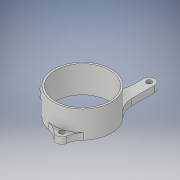
# Autodesk Inventor part: DPLX_P020_Camera Shroud Base_RevA
Saved by Autodesk Inventor 2018 (Build 220112000, 112)
## iProperties
Created: 2018-06-25
Part Number: DPLX_P020_Camera Shroud Base_RevA
Material: Generic
Document SubType Name: Modeling
Designer: Dplxuser
Density: 1 g/cm^3
Appearance: Default
Mass: 2.54454 g
Surface Area: 42.3669 cm^2
Volume: 2.54454 cm^3
Author: Dplxuser
Autodesk Inventor part; units mm, degrees
ref_plane "YZ Plane" through (0, 0, 0) normal (1, 0, 0) x (0, 1, 0)
ref_plane "XZ Plane" through (0, 0, 0) normal (0, 1, 0) x (-1, 0, 0)
ref_plane "XY Plane" through (0, 0, 0) normal (0, 0, 1) x (1, 0, 0)
sketch "Sketch2" plane through (0, 0, 0) normal (0, 1, 0) x (-1, 0, 0)
  circle A0 centre (-4.7625, 13.0048) radius 1.524 construction
  circle A1 centre (-25.3436, 13.0048) radius 6.35 construction
  circle A2 centre (-31.0168, 30.7721) radius 1.524 construction
  circle A3 centre (-31.0168, -20.6375) radius 1.524 construction
  line L0 (-38.1807, -25.4) -> (-38.1807, 35.5346) construction
  line L1 (-23.8528, -25.4) -> (-38.1807, -25.4) construction
  line L2 (-23.8528, 0) -> (-23.8528, -25.4) construction
  line L3 (0, 0) -> (-23.8528, 0) construction
  line L4 (0, 26.0096) -> (0, 0) construction
  line L5 (-23.8528, 26.0096) -> (0, 26.0096) construction
  line L6 (-23.8528, 26.0096) -> (-23.8528, 35.5346) construction
  line L7 (-38.1807, 35.5346) -> (-23.8528, 35.5346) construction
  point P0 (-23.8528, 13.0048)
  dimension "d3" = 3.048
  dimension "d4" = 12.7
  dimension "d5" = 90
  dimension "d6" = 23.8528
  dimension "d7" = 38.1807
  dimension "d8" = 26.0096
  dimension "d9" = 25.4
  dimension "d10" = 35.5346
  dimension "d11" = 0
  dimension "d12" = 0
  dimension "d13" = 23.8528
  dimension "d14" = 4.7625
  dimension "d15" = 13.0048
  dimension "d16" = 23.8528
  dimension "d17" = 13.0048
  dimension "d18" = 25.3436
  dimension "d19" = 13.0048
  dimension "d20" = 31.0167
  dimension "d21" = 30.7721
  dimension "d22" = 31.0167
  dimension "d23" = 20.6375
  constraints: 16 end point, 5 parallel, 4 centre point, 2 equal radius, 1 horizontal, 1 vertical
  measures "d3" diameter of A0
  measures "d4" diameter of A1
  measures "d5" angle of L3 L2
  measures "d6" distance between parallel lines of L4 L6
  measures "d7" distance between parallel lines of L4 L0
  measures "d8" distance between parallel lines of L5 L3
  measures "d9" distance between parallel lines of L3 L1
  measures "d10" distance between parallel lines of L3 L7
  measures "d11" distance from line of point (0, 0) L4
  measures "d12" distance from line of point (0, 0) L3
  measures "d13" distance from line of point (0, 0) L2
  measures "d14" distance from line of A0.centre L4
  measures "d15" distance from line of A0.centre L3
  measures "d16" distance from line of point (-23.853, 13.005) L4
  measures "d17" distance from line of point (-23.853, 13.005) L3
  measures "d18" distance from line of A1.centre L4
  measures "d19" distance from line of A1.centre L3
  measures "d20" distance from line of A2.centre L4
  measures "d21" distance from line of A2.centre L3
  measures "d22" distance from line of A3.centre L4
  measures "d23" distance from line of A3.centre L3
sketch "Sketch3" plane through (0, 0, 0) normal (0, 1, 0) x (-1, 0, 0)
  circle A0 centre (-25.3436, 13.0048) radius 15.875
  circle A1 centre (-31.0168, 30.7721) radius 1.524
  circle A2 centre (-4.7625, 13.0048) radius 1.524
  circle A3 centre (-31.0168, -20.6375) radius 1.524
  line L0 (-31.0168, 30.7721) -> (-31.0168, -20.6375) construction
  line L1 (-4.7625, 13.0048) -> (-31.0168, 13.0048) construction
  line L2 (-4.7625, 13.0048) -> (-3.2385, 13.0048) construction
  line L3 (-3.2385, 13.0048) -> (-3.2385, 32.2961) construction
  line L4 (-3.2385, 32.2961) -> (-31.0168, 32.2961) construction
  line L5 (-3.2385, 13.0048) -> (-3.2385, -22.1615) construction
  line L6 (-3.2385, -22.1615) -> (-31.0168, -22.1615) construction
  line L7 (-32.5408, 30.7721) -> (-32.5408, -22.1615) construction
  line L8 (-32.5408, -22.1615) -> (-31.0168, -22.1615) construction
  line L9 (-31.0168, 32.2961) -> (-32.5408, 32.2961) construction
  line L10 (-32.5408, 32.2961) -> (-32.5408, 30.7721) construction
  line L11 (-31.0168, 42.8789) -> (7.3443, 42.8789) construction
  line L12 (7.3443, 42.8789) -> (7.3443, 13.0048) construction
  line L13 (7.3443, 13.0048) -> (7.3443, -32.7443) construction
  line L14 (7.3443, -32.7443) -> (-15.7768, -32.7443) construction
  line L15 (-15.7768, -32.7443) -> (-27.8836, -32.7443) construction
  line L16 (-43.1236, 30.7721) -> (-43.1236, 42.8789) construction
  line L17 (-43.1236, 42.8789) -> (-31.0168, 42.8789) construction
  line L18 (-25.3436, 13.0048) -> (-35.5036, 13.0048) construction
  arc A4 (-25.3436, -2.8702) -> (-25.3436, 28.8798) centre (-25.3436, 13.0048) ccw
  line L19 (-27.8836, -32.7443) -> (-27.8836, -2.8702) construction
  line L20 (-43.1236, 28.8798) -> (-43.1236, 30.7721) construction
  line L21 (-34.3188, 30.7721) -> (-34.3188, 27.314)
  line L22 (-34.3188, -1.3044) -> (-34.3188, -20.6375)
  circle A5 centre (-25.3436, 13.0048) radius 16.891
  line L23 (-4.7625, 13.0048) -> (-25.3436, 13.0048) construction
  line L24 (-4.7625, 16.3068) -> (-8.7785, 16.3068)
  line L25 (-8.7785, 9.7028) -> (-4.7625, 9.7028)
  arc A6 (-4.7625, 9.7028) -> (-4.7625, 16.3068) centre (-4.7625, 13.0048) ccw
  line L26 (-31.0168, -20.6375) -> (-31.0168, 13.0048) construction
  line L27 (-27.7148, -20.6375) -> (-27.7148, -3.7189)
  line L28 (-34.3188, -1.3044) -> (-34.3188, -20.6375)
  arc A7 (-34.3188, -20.6375) -> (-27.7148, -20.6375) centre (-31.0168, -20.6375) ccw
  line L29 (-31.0168, 30.7721) -> (-31.0168, 13.0048) construction
  line L30 (-34.3188, 30.7721) -> (-34.3188, 27.314)
  arc A8 (-27.7148, 30.7721) -> (-34.3188, 30.7721) centre (-31.0168, 30.7721) ccw
  line L31 (-27.7148, 29.7285) -> (-27.7148, 30.7721)
  arc A9 (-30.2144, -23.8405) -> (-1.4605, 13.0048) centre (-39.4443, 13.0048) ccw construction
  arc A10 (-1.4605, 13.0048) -> (-32.2443, 33.8374) centre (-23.9015, 13.0048) ccw construction
  point P0 (0, 0)
  point P1 (-30.4236, 13.0048)
  point P2 (-15.053, 13.0048)
  point P3 (-31.0168, -3.8163)
  point P4 (-31.0168, 21.8885)
  dimension "d26" = 3.048
  dimension "d27" = 3.048
  dimension "d24" = 31.75
  dimension "d25" = 3.048
  dimension "d32" = 10.16
  dimension "d36" = 1.778
  dimension "d38" = 1.778
  dimension "d40" = 1.016
  dimension "d44" = 6.604
  dimension "d45" = 4.016
  constraints: 72 end point, 23 point on circle, 12 tangent, 10 perpendicular, 9 centre point, 6 vertical, 5 coincident, 4 midpoint, 3 collinear, 3 parallel, 2 horizontal, 2 point on line, 1 concentric, 1 horizontal alignment, 1 vertical alignment, 9 other
  measures "d24" diameter of A0
  measures "d25" diameter of A1
  measures "d32" distance of L18.start L18.end
  measures "d36" distance from line of L7.start L21
  measures "d38" distance between parallel lines of L7 L22
  measures "d40" radial gap between concentric circles of A4 A5
  measures "d44" distance between parallel lines of L25 L24
  measures "d45" distance of L25.start L25.end
extrude "Extrusion1" add sketch "Sketch3" along normal blind 15.875 contours A5
extrude "Extrusion2" add sketch "Sketch3" along normal blind 3.81 contours A8 L31 A5 L21 | A5 L27 A7 L22 | L24 A6 L25 A5
fillet "Fillet1" radius 12.7 6 edges at (27.7148, 1.905, 29.7285) (34.3188, 1.905, 27.314) (34.3188, 1.905, -1.3044) (8.7785, 1.905, 9.7028) (27.7148, 1.905, -3.7189) (8.7785, 1.905, 16.3068)
body "Solid1"
